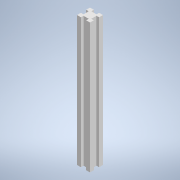
# Autodesk Inventor part: wysiegnik
Saved by Autodesk Inventor 2021 (Build 250183000, 183)
## iProperties
Created: 2021-06-18
Part Number: wysiegnik
Material: Ogólny
Document SubType Name: Modeling
Designer: Wojciech Wołczek
Density: 1 g/cm^3
Appearance: Domyślna
Author: Wojciech Wołczek
Autodesk Inventor part; units mm, degrees
ref_plane "YZ Plane" through (0, 0, 0) normal (1, 0, 0) x (0, 1, 0)
ref_plane "XZ Plane" through (0, 0, 0) normal (0, 1, 0) x (-1, 0, 0)
ref_plane "XY Plane" through (0, 0, 0) normal (0, 0, 1) x (1, 0, 0)
sketch "Szkic1" plane through (0, 0, 0) normal (0, 1, 0) x (-1, 0, 0)
  line L0 (-25, -25) -> (25, -25)
  line L1 (25, -25) -> (25, 25)
  line L2 (-25, 25) -> (-25, -25)
  line L3 (-25, -25) -> (25, 25) construction
  line L4 (25, -25) -> (-25, 25) construction
  line L5 (10, 25) -> (-10, 25)
  line L6 (-10, 25) -> (-10, 15)
  line L7 (-10, 15) -> (10, 15)
  line L8 (10, 15) -> (10, 25)
  line L9 (-15, -10) -> (-15, 10)
  line L10 (-15, 10) -> (-25, 10)
  line L11 (-25, -10) -> (-15, -10)
  line L12 (10, -15) -> (-10, -15)
  line L13 (-10, -15) -> (-10, -25)
  line L14 (10, -25) -> (10, -15)
  line L15 (15, 10) -> (15, -10)
  line L16 (15, -10) -> (25, -10)
  line L17 (25, 10) -> (15, 10)
  line L18 (25, 25) -> (10, 25)
  line L19 (-10, 25) -> (-25, 25)
  point P0 (0, 0)
  dimension "d0" = 50
  dimension "d1" = 50
  dimension "d3" = 10
  dimension "d7" = 360
  constraints: 40 end point, 5 parallel, 2 horizontal, 2 midpoint, 2 perpendicular, 29 other
  measures "d0" distance of L2.start L1.end
  measures "d1" distance of L1.end L0.end
  measures "d3" distance of L6.end L5.end
extrude "Wyciągnięcie proste1" add sketch "Szkic1" along normal blind 500 contours L2 L11 L9 L10 L19 L6 L7 L8 L18 L1 L17 L15 L16 L0 L14 L12 L13
